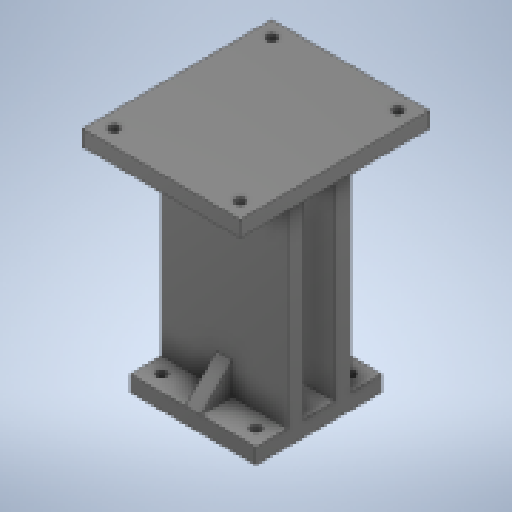
# Autodesk Inventor part: lidar
Saved by Autodesk Inventor 2026.2 (Build 302298010, 298A)
## iProperties
Created: 2026-05-04
Part Number: lidar
Material: ABS Plastic
Document SubType Name: Modeling
Designer: chris
Density: 1.06 g/cm^3
Appearance: Smooth - White
Author: chris
Autodesk Inventor part; units mm, degrees
sketch "Sketch1" plane through (0, 0, 0) normal (0, 1, 0) x (-1, 0, 0)
  line L0 (40, 40) -> (-40, 40)
  line L1 (-40, 40) -> (-40, -40)
  line L2 (-40, -40) -> (40, -40)
  line L3 (40, -40) -> (40, 40)
  line L4 (40, 40) -> (-40, -40) construction
  line L5 (-40, 40) -> (40, -40) construction
  point P0 (0, 0)
  dimension "d0" = 80
  dimension "d1" = 80
  constraints: 12 end point, 2 midpoint, 2 parallel, 1 horizontal, 1 perpendicular
  measures "d0" distance of L2.end L1.end
  measures "d1" distance of L1.end L0.end
extrude "Extrusion1" add sketch "Sketch1" along normal blind 10
sketch "Sketch2" plane through (0, 10, 0) normal (0, 1, 0) x (1, 0, 0)
  circle A0 centre (30, 30) radius 3.1
  circle A1 centre (30, -30) radius 3.1
  circle A2 centre (-30, -30) radius 3.1
  circle A3 centre (-30, 30) radius 3.1
  point P0 (0, 0)
  dimension "d4" = 6.2
  dimension "d5" = 6.2
  dimension "d6" = 6.2
  dimension "d7" = 6.2
  dimension "d8" = 30
  dimension "d9" = 30
  dimension "d10" = 30
  dimension "d11" = 30
  dimension "d12" = 30
  dimension "d13" = 30
  dimension "d14" = 30
  dimension "d15" = 30
  constraints: 4 centre point
  measures "d4" diameter of A0
  measures "d5" diameter of A1
  measures "d6" diameter of A2
  measures "d7" diameter of A3
  measures "d8" horizontal distance of A0.centre point (0, 0)
  measures "d9" horizontal distance of A3.centre point (0, 0)
  measures "d10" horizontal distance of point (0, 0) A2.centre
  measures "d11" horizontal distance of point (0, 0) A1.centre
  measures "d12" horizontal distance of A3.centre point (0, 0)
  measures "d13" horizontal distance of point (0, 0) A0.centre
  measures "d14" horizontal distance of point (0, 0) A2.centre
  measures "d15" horizontal distance of point (0, 0) A1.centre
extrude "Extrusion2" cut sketch "Sketch2" against normal blind 10
sketch "Sketch3" plane through (0, 10, 0) normal (0, 1, 0) x (1, 0, 0)
  line L0 (40, 10) -> (-40, 10)
  line L1 (-40, 10) -> (-40, 20)
  line L2 (-40, 20) -> (40, 20)
  line L3 (40, 20) -> (40, 10)
  line L4 (40, 10) -> (-40, 20) construction
  line L5 (-40, 10) -> (40, 20) construction
  line L6 (40, -20) -> (-40, -20)
  line L7 (-40, -20) -> (-40, -10)
  line L8 (-40, -10) -> (40, -10)
  line L9 (40, -10) -> (40, -20)
  line L10 (40, -20) -> (-40, -10) construction
  line L11 (-40, -20) -> (40, -10) construction
  line L12 (-40, 40) -> (-40, -40) projected
  line L13 (40, -40) -> (40, 40) projected
  line L14 (40, 40) -> (-40, 40) projected
  line L15 (-40, -40) -> (40, -40) projected
  point P0 (0, 0)
  point P1 (0, 15)
  point P2 (0, -15)
  dimension "d19" = 10
  dimension "d20" = 10
  dimension "d21" = 20
  dimension "d22" = 20
  constraints: 24 end point, 4 collinear, 4 midpoint, 4 parallel, 2 horizontal, 2 perpendicular
  measures "d19" distance of L6.end L7.end
  measures "d20" distance of L0.end L1.end
  measures "d21" distance between parallel lines of L14 L2
  measures "d22" distance between parallel lines of L15 L6
extrude "Extrusion3" add sketch "Sketch3" along normal blind 130 contours L0 L1 L2 L3 | L9 L6 L7 L8
sketch "Sketch4" plane through (0, 10, 0) normal (0, 1, 0) x (1, 0, 0)
  line L0 (20, -10) -> (-20, -10)
  line L1 (-20, -10) -> (-20, 10)
  line L2 (-20, 10) -> (20, 10)
  line L3 (20, 10) -> (20, -10)
  line L4 (20, -10) -> (-20, 10) construction
  line L5 (-20, -10) -> (20, 10) construction
  line L6 (-40, 10) -> (40, 10) projected
  point P0 (0, 0)
  dimension "d25" = 40
  constraints: 12 end point, 2 midpoint, 2 parallel, 1 collinear, 1 horizontal, 1 perpendicular
  measures "d25" distance of L1.end L2.end
extrude "Extrusion4" cut sketch "Sketch4" against normal blind 10
sketch "Sketch5" plane through (0, 140, 0) normal (0, 1, 0) x (1, 0, 0)
  line L0 (50, -60) -> (-50, -60)
  line L1 (-50, -60) -> (-50, 60)
  line L2 (-50, 60) -> (50, 60)
  line L3 (50, 60) -> (50, -60)
  line L4 (50, -60) -> (-50, 60) construction
  line L5 (-50, -60) -> (50, 60) construction
  point P0 (0, 0)
  dimension "d28" = 100
  dimension "d29" = 120
  constraints: 12 end point, 2 midpoint, 2 parallel, 1 horizontal, 1 perpendicular
  measures "d28" distance of L1.end L2.end
  measures "d29" distance of L0.end L1.end
extrude "Extrusion5" add sketch "Sketch5" along normal blind 10
sketch "Sketch6" plane through (0, 150, 0) normal (0, 1, 0) x (1, 0, 0)
  circle A0 centre (-40, 50) radius 3.1
  circle A1 centre (40, 50) radius 3.1
  circle A2 centre (40, -50) radius 3.1
  circle A3 centre (-40, -50) radius 3.1
  point P0 (0, 0)
  dimension "d32" = 6.2
  dimension "d33" = 6.2
  dimension "d34" = 6.2
  dimension "d35" = 6.2
  dimension "d36" = 50
  dimension "d37" = 50
  dimension "d38" = 50
  dimension "d39" = 50
  dimension "d40" = 40
  dimension "d41" = 40
  dimension "d42" = 40
  dimension "d43" = 40
  constraints: 4 centre point
  measures "d32" diameter of A0
  measures "d33" diameter of A1
  measures "d34" diameter of A2
  measures "d35" diameter of A3
  measures "d36" vertical distance of A0.centre point (0, 0)
  measures "d37" vertical distance of A3.centre point (0, 0)
  measures "d38" vertical distance of point (0, 0) A2.centre
  measures "d39" vertical distance of A1.centre point (0, 0)
  measures "d40" horizontal distance of point (0, 0) A1.centre
  measures "d41" horizontal distance of A0.centre point (0, 0)
  measures "d42" horizontal distance of point (0, 0) A3.centre
  measures "d43" horizontal distance of point (0, 0) A2.centre
extrude "Extrusion6" cut sketch "Sketch6" against normal blind 10
ref_plane "Work Plane1" through (0, 0, 40) normal (1, 0, 0) x (0, 0, -1)
sketch "Sketch7" plane through (0, 0, 40) normal (1, 0, 0) x (0, 0, -1)
  line L0 (80, 10) -> (60, 10)
  line L1 (60, 10) -> (60, 30)
  line L2 (60, 10) -> (80, 10) projected
  line L3 (60, 10) -> (60, 140) projected
  line L4 (60, 30) -> (80, 10)
  point P0 (40, 0)
  dimension "d47" = 20
  dimension "d48" = 20
  constraints: 6 end point, 2 collinear, 1 horizontal, 1 perpendicular
  measures "d47" distance of L0.start L0.end
  measures "d48" distance of L0.end L1.end
extrude "Extrusion7" add sketch "Sketch7" along normal mid plane 10
ref_plane "Work Plane2" through (0, 75, 0) normal (0, -1, 0) x (1, 0, 0)
mirror "Mirror1" about plane through (0, 75, 0) normal (0, -1, 0) of "Extrusion7"
ref_plane "Work Plane3" through (40, 0, 0) normal (0, 0, -1) x (-1, 0, 0)
mirror "Mirror2" about plane through (40, 0, 0) normal (0, 0, -1) of "Extrusion7", "Mirror1"
body "Solid1"
